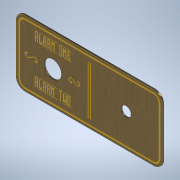
# Autodesk Inventor part: EW_MessingplatteBedienelemente
Saved by Autodesk Inventor 2020 (Build 240168000, 168)
## iProperties
Created: 2020-06-21
Part Number: EW_MessingplatteBedienelemente
Material: Messing
Document SubType Name: Modeling
Designer: Johannes
Density: 8.49 g/cm^3
Appearance: Messing - satiniert 1
Author: Johannes
Autodesk Inventor part; units mm, degrees
ref_plane "YZ Plane" through (0, 0, 0) normal (1, 0, 0) x (0, 1, 0)
ref_plane "XZ Plane" through (0, 0, 0) normal (0, 1, 0) x (-1, 0, 0)
ref_plane "XY Plane" through (0, 0, 0) normal (0, 0, 1) x (1, 0, 0)
sketch "Skizze2" plane through (0, 0, 0) normal (0, 0, 1) x (1, 0, 0)
  line L0 (-50, -22.5) -> (50, -22.5)
  line L1 (50, -22.5) -> (50, 22.5)
  line L2 (50, 22.5) -> (-50, 22.5)
  line L3 (-50, 22.5) -> (-50, -22.5)
  line L4 (-50, -22.5) -> (50, 22.5) construction
  line L5 (50, -22.5) -> (-50, 22.5) construction
  point P0 (0, 0)
  dimension "d0" = 100
  dimension "d1" = 45
  constraints: 12 end point, 2 midpoint, 2 parallel, 1 horizontal, 1 perpendicular
  measures "d0" distance of L2.end L1.end
  measures "d1" distance of L1.end L0.end
extrude "Extrusion1" add sketch "Skizze2" along normal blind 0.8
fillet "Rundung1" radius 6 4 edges at (-50, 22.5, 0.4) (50, 22.5, 0.4) (50, -22.5, 0.4) (-50, -22.5, 0.4)
sketch "Skizze3" plane through (0, 0, 0.8) normal (0, 0, 1) x (1, 0, 0)
  line L0 (-50, 22.5) -> (50, 22.5) construction
  line L1 (50, 22.5) -> (50, -22.6939) construction
  line L2 (50, -22.6939) -> (-50, -22.6939) construction
  line L3 (-50, -22.6939) -> (-50, 22.5) construction
  line L4 (-50, 16.5) -> (-50, -16.5) projected
  line L5 (44, 22.5) -> (-44, 22.5) projected
  point P0 (0, 0)
  dimension "d6" = 100
  constraints: 2 collinear, 2 other
  measures "d6" distance of L0.start L0.end
decal "Aufkleber1"
sketch "Skizze4" plane through (0, 0, 0.8) normal (0, 0, 1) x (1, 0, 0)
  circle A0 centre (-25, 0) radius 6
  line L0 (44, 22.5) -> (-44, 22.5) projected
  line L1 (-50, 16.5) -> (-50, -16.5) projected
  circle A1 centre (25, 0) radius 3.5
  line L2 (50, -16.5) -> (50, 16.5) projected
  point P0 (0, 0)
  dimension "d10" = 22.5
  dimension "d11" = 25
  dimension "d12" = 12
  dimension "d15" = 25
  dimension "d16" = 7
  constraints: 2 centre point, 1 horizontal alignment
  measures "d10" distance from line of A0.centre L0
  measures "d11" distance from line of L1 A0.centre
  measures "d12" diameter of A0
  measures "d15" distance from line of L2 A1.centre
  measures "d16" diameter of A1
extrude "Extrusion2" cut sketch "Skizze4" against normal through all
